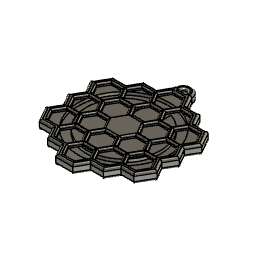
Base-v02 v3 (Autodesk Fusion 360 design; units mm, degrees)
Autodesk Fusion 360 part; units mm, degrees
note: some values were not read from the file. Set by a fixed rule: which sketch regions a step uses.
(part 1 of 2)
sketch "Skizze1" plane through (0, 0, 0) normal (0, 0, 1) x (1, 0, 0)
  line L0 (2.1651, -11.25) -> (4.3301, -7.5) construction
  line L1 (4.3301, -7.5) -> (2.1651, -3.75) construction
  line L2 (2.1651, -3.75) -> (-2.1651, -3.75) construction
  line L3 (-2.1651, -3.75) -> (-4.3301, -7.5) construction
  line L4 (-4.3301, -7.5) -> (-2.1651, -11.25) construction
  line L5 (-2.1651, -11.25) -> (2.1651, -11.25) construction
  line L6 (-2.1651, -3.75) -> (-4.3301, 0) construction
  line L7 (-4.3301, 0) -> (-8.6603, 0) construction
  line L8 (-8.6603, 0) -> (-10.8253, -3.75) construction
  line L9 (-10.8253, -3.75) -> (-8.6603, -7.5) construction
  line L10 (-8.6603, -7.5) -> (-4.3301, -7.5) construction
  line L11 (-4.3301, -7.5) -> (-2.1651, -3.75) construction
  line L12 (-4.3301, -7.5) -> (-8.6603, -7.5) construction
  line L13 (-8.6603, -7.5) -> (-10.8253, -11.25) construction
  line L14 (-10.8253, -11.25) -> (-8.6603, -15) construction
  line L15 (-8.6603, -15) -> (-4.3301, -15) construction
  line L16 (-4.3301, -15) -> (-2.1651, -11.25) construction
  line L17 (-2.1651, -11.25) -> (-4.3301, -7.5) construction
  line L18 (10.8253, -11.25) -> (8.6603, -7.5) construction
  line L19 (8.6603, -7.5) -> (4.3301, -7.5) construction
  line L20 (4.3301, -7.5) -> (2.1651, -11.25) construction
  line L21 (2.1651, -11.25) -> (4.3301, -15) construction
  line L22 (4.3301, -15) -> (8.6603, -15) construction
  line L23 (8.6603, -15) -> (10.8253, -11.25) construction
  line L24 (10.8253, -3.75) -> (8.6603, 0) construction
  line L25 (8.6603, 0) -> (4.3301, 0) construction
  line L26 (4.3301, 0) -> (2.1651, -3.75) construction
  line L27 (2.1651, -3.75) -> (4.3301, -7.5) construction
  line L28 (4.3301, -7.5) -> (8.6603, -7.5) construction
  line L29 (8.6603, -7.5) -> (10.8253, -3.75) construction
  line L30 (17.3205, 0) -> (15.1554, 3.75) construction
  line L31 (15.1554, 3.75) -> (10.8253, 3.75) construction
  line L32 (10.8253, 3.75) -> (8.6603, 0) construction
  line L33 (8.6603, 0) -> (10.8253, -3.75) construction
  line L34 (10.8253, -3.75) -> (15.1554, -3.75) construction
  line L35 (15.1554, -3.75) -> (17.3205, 0) construction
  line L36 (8.6603, -7.5) -> (10.8253, -11.25) construction
  line L37 (10.8253, -11.25) -> (15.1554, -11.25) construction
  line L38 (15.1554, -11.25) -> (17.3205, -7.5) construction
  line L39 (17.3205, -7.5) -> (15.1554, -3.75) construction
  line L40 (15.1554, -3.75) -> (10.8253, -3.75) construction
  line L41 (10.8253, -3.75) -> (8.6603, -7.5) construction
  line L42 (-4.3301, 0) -> (-2.1651, -3.75) construction
  line L43 (-2.1651, -3.75) -> (2.1651, -3.75) construction
  line L44 (2.1651, -3.75) -> (4.3301, 0) construction
  line L45 (4.3301, 0) -> (2.1651, 3.75) construction
  line L46 (2.1651, 3.75) -> (-2.1651, 3.75) construction
  line L47 (-2.1651, 3.75) -> (-4.3301, 0) construction
  line L48 (-8.6603, -22.5) -> (-4.3301, -22.5) construction
  line L49 (-4.3301, -22.5) -> (-2.1651, -18.75) construction
  line L50 (-2.1651, -18.75) -> (-4.3301, -15) construction
  line L51 (-4.3301, -15) -> (-8.6603, -15) construction
  line L52 (-8.6603, -15) -> (-10.8253, -18.75) construction
  line L53 (-10.8253, -18.75) -> (-8.6603, -22.5) construction
  line L54 (8.6603, -30) -> (10.8253, -26.25) construction
  line L55 (10.8253, -26.25) -> (8.6603, -22.5) construction
  line L56 (8.6603, -22.5) -> (4.3301, -22.5) construction
  line L57 (4.3301, -22.5) -> (2.1651, -26.25) construction
  line L58 (2.1651, -26.25) -> (4.3301, -30) construction
  line L59 (4.3301, -30) -> (8.6603, -30) construction
  line L60 (2.1651, -26.25) -> (4.3301, -22.5) construction
  line L61 (4.3301, -22.5) -> (2.1651, -18.75) construction
  line L62 (2.1651, -18.75) -> (-2.1651, -18.75) construction
  line L63 (-2.1651, -18.75) -> (-4.3301, -22.5) construction
  line L64 (-4.3301, -22.5) -> (-2.1651, -26.25) construction
  line L65 (-2.1651, -26.25) -> (2.1651, -26.25) construction
  line L66 (23.8157, -11.25) -> (21.6506, -7.5) construction
  line L67 (21.6506, -7.5) -> (17.3205, -7.5) construction
  line L68 (17.3205, -7.5) -> (15.1554, -11.25) construction
  line L69 (15.1554, -11.25) -> (17.3205, -15) construction
  line L70 (17.3205, -15) -> (21.6506, -15) construction
  line L71 (21.6506, -15) -> (23.8157, -11.25) construction
  line L72 (10.8253, -18.75) -> (8.6603, -15) construction
  line L73 (8.6603, -15) -> (4.3301, -15) construction
  line L74 (4.3301, -15) -> (2.1651, -18.75) construction
  line L75 (2.1651, -18.75) -> (4.3301, -22.5) construction
  line L76 (4.3301, -22.5) -> (8.6603, -22.5) construction
  line L77 (8.6603, -22.5) -> (10.8253, -18.75) construction
  line L78 (15.1554, -18.75) -> (10.8253, -18.75) construction
  line L79 (10.8253, -18.75) -> (8.6603, -22.5) construction
  line L80 (8.6603, -22.5) -> (10.8253, -26.25) construction
  line L81 (10.8253, -26.25) -> (15.1554, -26.25) construction
  line L82 (15.1554, -26.25) -> (17.3205, -22.5) construction
  line L83 (17.3205, -22.5) -> (15.1554, -18.75) construction
  line L84 (8.6603, 7.5) -> (4.3301, 7.5) construction
  line L85 (4.3301, 7.5) -> (2.1651, 3.75) construction
  line L86 (2.1651, 3.75) -> (4.3301, 0) construction
  line L87 (4.3301, 0) -> (8.6603, 0) construction
  line L88 (8.6603, 0) -> (10.8253, 3.75) construction
  line L89 (10.8253, 3.75) -> (8.6603, 7.5) construction
  line L90 (15.1554, -11.25) -> (10.8253, -11.25) construction
  line L91 (10.8253, -11.25) -> (8.6603, -15) construction
  line L92 (8.6603, -15) -> (10.8253, -18.75) construction
  line L93 (10.8253, -18.75) -> (15.1554, -18.75) construction
  line L94 (15.1554, -18.75) -> (17.3205, -15) construction
  line L95 (17.3205, -15) -> (15.1554, -11.25) construction
  line L96 (21.6506, 0) -> (17.3205, 0) construction
  line L97 (17.3205, 0) -> (15.1554, -3.75) construction
  line L98 (15.1554, -3.75) -> (17.3205, -7.5) construction
  line L99 (17.3205, -7.5) -> (21.6506, -7.5) construction
  line L100 (21.6506, -7.5) -> (23.8157, -3.75) construction
  line L101 (23.8157, -3.75) -> (21.6506, 0) construction
  line L102 (2.1651, -18.75) -> (4.3301, -15) construction
  line L103 (4.3301, -15) -> (2.1651, -11.25) construction
  line L104 (2.1651, -11.25) -> (-2.1651, -11.25) construction
  line L105 (-2.1651, -11.25) -> (-4.3301, -15) construction
  line L106 (-4.3301, -15) -> (-2.1651, -18.75) construction
  line L107 (-2.1651, -18.75) -> (2.1651, -18.75) construction
  line L108 (23.8157, -18.75) -> (21.6506, -15) construction
  line L109 (21.6506, -15) -> (17.3205, -15) construction
  line L110 (17.3205, -15) -> (15.1554, -18.75) construction
  line L111 (15.1554, -18.75) -> (17.3205, -22.5) construction
  line L112 (17.3205, -22.5) -> (21.6506, -22.5) construction
  line L113 (21.6506, -22.5) -> (23.8157, -18.75) construction
  line L114 (4.6765, 0.6) -> (8.3138, 0.6)
  line L115 (8.3138, 0.6) -> (10.1325, 3.75)
  line L116 (10.1325, 3.75) -> (8.3138, 6.9)
  line L117 (8.3138, 6.9) -> (4.6765, 6.9)
  line L118 (4.6765, 6.9) -> (2.8579, 3.75)
  line L119 (2.8579, 3.75) -> (4.6765, 0.6)
  line L120 (14.809, -3.15) -> (16.6277, 0)
  line L121 (16.6277, 0) -> (14.809, 3.15)
  line L122 (14.809, 3.15) -> (11.1717, 3.15)
  line L123 (11.1717, 3.15) -> (9.3531, 0)
  line L124 (9.3531, 0) -> (11.1717, -3.15)
  line L125 (11.1717, -3.15) -> (14.809, -3.15)
  line L126 (21.3042, -6.9) -> (23.1229, -3.75)
  line L127 (23.1229, -3.75) -> (21.3042, -0.6)
  line L128 (21.3042, -0.6) -> (17.6669, -0.6)
  line L129 (17.6669, -0.6) -> (15.8483, -3.75)
  line L130 (15.8483, -3.75) -> (17.6669, -6.9)
  line L131 (17.6669, -6.9) -> (21.3042, -6.9)
  line L132 (14.809, -10.65) -> (16.6277, -7.5)
  line L133 (16.6277, -7.5) -> (14.809, -4.35)
  line L134 (14.809, -4.35) -> (11.1717, -4.35)
  line L135 (11.1717, -4.35) -> (9.3531, -7.5)
  line L136 (9.3531, -7.5) -> (11.1717, -10.65)
  line L137 (11.1717, -10.65) -> (14.809, -10.65)
  line L138 (15.8483, -11.25) -> (17.6669, -14.4)
  line L139 (17.6669, -14.4) -> (21.3042, -14.4)
  line L140 (21.3042, -14.4) -> (23.1229, -11.25)
  line L141 (23.1229, -11.25) -> (21.3042, -8.1)
  line L142 (21.3042, -8.1) -> (17.6669, -8.1)
  line L143 (17.6669, -8.1) -> (15.8483, -11.25)
  line L144 (11.1717, -18.15) -> (14.809, -18.15)
  line L145 (14.809, -18.15) -> (16.6277, -15)
  line L146 (16.6277, -15) -> (14.809, -11.85)
  line L147 (14.809, -11.85) -> (11.1717, -11.85)
  line L148 (11.1717, -11.85) -> (9.3531, -15)
  line L149 (9.3531, -15) -> (11.1717, -18.15)
  line L150 (-1.8187, -10.65) -> (1.8187, -10.65)
  line L151 (1.8187, -10.65) -> (3.6373, -7.5)
  line L152 (3.6373, -7.5) -> (1.8187, -4.35)
  line L153 (1.8187, -4.35) -> (-1.8187, -4.35)
  line L154 (-1.8187, -4.35) -> (-3.6373, -7.5)
  line L155 (-3.6373, -7.5) -> (-1.8187, -10.65)
  line L156 (-1.8187, -3.15) -> (1.8187, -3.15)
  line L157 (1.8187, -3.15) -> (3.6373, 0)
  line L158 (3.6373, 0) -> (1.8187, 3.15)
  line L159 (1.8187, 3.15) -> (-1.8187, 3.15)
  line L160 (-1.8187, 3.15) -> (-3.6373, 0)
  line L161 (-3.6373, 0) -> (-1.8187, -3.15)
  line L162 (-8.3138, -6.9) -> (-4.6765, -6.9)
  line L163 (-4.6765, -6.9) -> (-2.8579, -3.75)
  line L164 (-2.8579, -3.75) -> (-4.6765, -0.6)
  line L165 (-4.6765, -0.6) -> (-8.3138, -0.6)
  line L166 (-8.3138, -0.6) -> (-10.1325, -3.75)
  line L167 (-10.1325, -3.75) -> (-8.3138, -6.9)
  line L168 (-0.0476, -15) -> (-0.0238, -15.0412)
  line L169 (-0.0238, -15.0412) -> (0.0238, -15.0412)
  line L170 (0.0238, -15.0412) -> (0.0476, -15)
  line L171 (0.0476, -15) -> (0.0238, -14.9588)
  line L172 (0.0238, -14.9588) -> (-0.0238, -14.9588)
  line L173 (-0.0238, -14.9588) -> (-0.0476, -15)
  line L174 (10.1325, -18.75) -> (8.3138, -15.6)
  line L175 (8.3138, -15.6) -> (4.6765, -15.6)
  line L176 (4.6765, -15.6) -> (2.8579, -18.75)
  line L177 (2.8579, -18.75) -> (4.6765, -21.9)
  line L178 (4.6765, -21.9) -> (8.3138, -21.9)
  line L179 (8.3138, -21.9) -> (10.1325, -18.75)
  line L180 (23.1229, -18.75) -> (21.3042, -15.6)
  line L181 (21.3042, -15.6) -> (17.6669, -15.6)
  line L182 (17.6669, -15.6) -> (15.8483, -18.75)
  line L183 (15.8483, -18.75) -> (17.6669, -21.9)
  line L184 (17.6669, -21.9) -> (21.3042, -21.9)
  line L185 (21.3042, -21.9) -> (23.1229, -18.75)
  line L186 (8.3138, -6.9) -> (10.1325, -3.75)
  line L187 (10.1325, -3.75) -> (8.3138, -0.6)
  line L188 (8.3138, -0.6) -> (4.6765, -0.6)
  line L189 (4.6765, -0.6) -> (2.8579, -3.75)
  line L190 (2.8579, -3.75) -> (4.6765, -6.9)
  line L191 (4.6765, -6.9) -> (8.3138, -6.9)
  line L192 (-4.6765, -21.9) -> (-2.8579, -18.75)
  line L193 (-2.8579, -18.75) -> (-4.6765, -15.6)
  line L194 (-4.6765, -15.6) -> (-8.3138, -15.6)
  line L195 (-8.3138, -15.6) -> (-10.1325, -18.75)
  line L196 (-10.1325, -18.75) -> (-8.3138, -21.9)
  line L197 (-8.3138, -21.9) -> (-4.6765, -21.9)
  line L198 (1.8187, -25.65) -> (3.6373, -22.5)
  line L199 (3.6373, -22.5) -> (1.8187, -19.35)
  line L200 (1.8187, -19.35) -> (-1.8187, -19.35)
  line L201 (-1.8187, -19.35) -> (-3.6373, -22.5)
  line L202 (-3.6373, -22.5) -> (-1.8187, -25.65)
  line L203 (-1.8187, -25.65) -> (1.8187, -25.65)
  line L204 (10.1325, -26.25) -> (8.3138, -23.1)
  line L205 (8.3138, -23.1) -> (4.6765, -23.1)
  line L206 (4.6765, -23.1) -> (2.8579, -26.25)
  line L207 (2.8579, -26.25) -> (4.6765, -29.4)
  line L208 (4.6765, -29.4) -> (8.3138, -29.4)
  line L209 (8.3138, -29.4) -> (10.1325, -26.25)
  line L210 (16.6277, -22.5) -> (14.809, -19.35)
  line L211 (14.809, -19.35) -> (11.1717, -19.35)
  line L212 (11.1717, -19.35) -> (9.3531, -22.5)
  line L213 (9.3531, -22.5) -> (11.1717, -25.65)
  line L214 (11.1717, -25.65) -> (14.809, -25.65)
  line L215 (14.809, -25.65) -> (16.6277, -22.5)
  line L216 (-1.8187, -18.15) -> (1.8187, -18.15)
  line L217 (1.8187, -18.15) -> (3.6373, -15)
  line L218 (3.6373, -15) -> (1.8187, -11.85)
  line L219 (1.8187, -11.85) -> (-1.8187, -11.85)
  line L220 (-1.8187, -11.85) -> (-3.6373, -15)
  line L221 (-3.6373, -15) -> (-1.8187, -18.15)
  line L222 (-8.3138, -14.4) -> (-4.6765, -14.4)
  line L223 (-4.6765, -14.4) -> (-2.8579, -11.25)
  line L224 (-2.8579, -11.25) -> (-4.6765, -8.1)
  line L225 (-4.6765, -8.1) -> (-8.3138, -8.1)
  line L226 (-8.3138, -8.1) -> (-10.1325, -11.25)
  line L227 (-10.1325, -11.25) -> (-8.3138, -14.4)
  line L228 (11.5181, 4.95) -> (9.3531, 8.7)
  line L229 (9.3531, 8.7) -> (3.6373, 8.7)
  line L230 (3.6373, 8.7) -> (1.4722, 4.95)
  line L231 (1.4722, 4.95) -> (-2.8579, 4.95)
  line L232 (-2.8579, 4.95) -> (-5.0229, 1.2)
  line L233 (-5.0229, 1.2) -> (-9.3531, 1.2)
  line L234 (-9.3531, 1.2) -> (-12.211, -3.75)
  line L235 (-12.211, -3.75) -> (-10.0459, -7.5)
  line L236 (-10.0459, -7.5) -> (-12.211, -11.25)
  line L237 (-12.211, -11.25) -> (-10.0459, -15)
  line L238 (-10.0459, -15) -> (-12.211, -18.75)
  line L239 (-12.211, -18.75) -> (-9.3531, -23.7)
  line L240 (-9.3531, -23.7) -> (-5.0229, -23.7)
  line L241 (-5.0229, -23.7) -> (-2.8579, -27.45)
  line L242 (-2.8579, -27.45) -> (1.4722, -27.45)
  line L243 (1.4722, -27.45) -> (3.6373, -31.2)
  line L244 (3.6373, -31.2) -> (9.3531, -31.2)
  line L245 (9.3531, -31.2) -> (11.5181, -27.45)
  line L246 (11.5181, -27.45) -> (15.8483, -27.45)
  line L247 (15.8483, -27.45) -> (18.0133, -23.7)
  line L248 (18.0133, -23.7) -> (22.3435, -23.7)
  line L249 (22.3435, -23.7) -> (25.2013, -18.75)
  line L250 (25.2013, -18.75) -> (23.0363, -15)
  line L251 (23.0363, -15) -> (25.2013, -11.25)
  line L252 (25.2013, -11.25) -> (23.0363, -7.5)
  line L253 (23.0363, -7.5) -> (25.2013, -3.75)
  line L254 (25.2013, -3.75) -> (22.3435, 1.2)
  line L255 (22.3435, 1.2) -> (18.0133, 1.2)
  line L256 (18.0133, 1.2) -> (15.8483, 4.95)
  line L257 (15.8483, 4.95) -> (11.5181, 4.95)
  arc A0 (9.3531, 8.7) -> (3.6373, 8.7) centre (6.4952, 8.7) ccw
  arc A1 (7.5531, 8.7) -> (5.4373, 8.7) centre (6.4952, 8.7) ccw
  point P0 (0, -7.5)
  point P1 (-6.4952, -3.75)
  point P2 (-6.4952, -11.25)
  point P3 (6.4952, -11.25)
  point P4 (6.4952, -3.75)
  point P5 (12.9904, 0)
  point P6 (12.9904, -7.5)
  point P7 (-6.4952, -18.75)
  point P8 (6.4952, -26.25)
  point P9 (0, -22.5)
  point P10 (19.4856, -11.25)
  point P11 (6.4952, -18.75)
  point P12 (12.9904, -22.5)
  point P13 (6.4952, 3.75)
  point P14 (12.9904, -15)
  point P15 (19.4856, -3.75)
  point P16 (0, -15)
  point P17 (19.4856, -18.75)
  point P18 (6.4952, 3.75)
  point P19 (12.9904, 0)
  point P20 (19.4856, -3.75)
  point P21 (12.9904, -7.5)
  point P22 (19.4856, -11.25)
  point P23 (12.9904, -15)
  point P24 (6.4952, -11.25)
  point P25 (0, -7.5)
  point P26 (-6.4952, -3.75)
  point P27 (-6.4952, -11.25)
  point P28 (0, -15)
  point P29 (6.4952, -18.75)
  point P30 (19.4856, -18.75)
  point P31 (6.4952, -3.75)
  point P32 (-6.4952, -18.75)
  point P33 (0, -22.5)
  point P34 (6.4952, -26.25)
  point P35 (12.9904, -22.5)
  point P36 (0, -15)
  point P37 (-6.4952, -11.25)
  point P38 (6.4952, 8.7)
  point P39 (6.4952, 6.9)
  dimension "d1" = 7.5
  dimension "d2" = 6.3
  dimension "d3" = 1.2
  dimension "d8" = 39.9
  dimension "d9" = -1.8
  constraint horizontal L2
  constraint equal L40 L45
  constraint equal L32 L45
  constraint equal L26 L40
  constraint equal L2 L40
  constraint equal L19 L40
  constraint equal L13 L46
  constraint equal L7 L46
  constraint equal L46 L103
  constraint equal L46 L55
  constraint equal L46 L50
  constraint equal L45 L61
  constraint equal L44 L67
  constraint equal L44 L73
  constraint equal L44 L79
  constraint equal L44 L85
  constraint equal L44 L91
  constraint equal L44 L97
  constraint horizontal L51
  constraint horizontal L46
  constraint horizontal L40
  constraint horizontal L31
  constraint horizontal L25
  constraint horizontal L7
  constraint horizontal L56
  constraint horizontal L104
  constraint horizontal L19
  constraint horizontal L96
  constraint horizontal L90
  constraint horizontal L84
  constraint horizontal L78
  constraint horizontal L73
  constraint horizontal L67
  constraint horizontal L62
  constraint midpoint L6 L42
  constraint midpoint L2 L43
  constraint midpoint L26 L44
  constraint midpoint L29 L41
  constraint midpoint L19 L28
  constraint midpoint L34 L40
  constraint midpoint L35 L97
  constraint midpoint L37 L90
  constraint midpoint L5 L104
  constraint midpoint L22 L73
  constraint horizontal L12
  constraint midpoint L10 L12
  constraint midpoint L25 L87
  constraint midpoint L15 L51
  constraint midpoint L62 L107
  constraint midpoint L56 L76
  constraint midpoint L78 L93
  constraint midpoint L67 L99
  constraint equal L46 L109
  constraint horizontal L109
  constraint midpoint L70 L109
  constraint coincident P18 P13
  constraint coincident P19 P5
  constraint coincident P20 P15
  constraint coincident P21 P6
  constraint coincident P22 P10
  constraint coincident P23 P14
  constraint coincident P24 P3
  constraint coincident P25 P0
  constraint coincident P26 P1
  constraint coincident P37 P27
  constraint coincident P36 P28
  constraint coincident P29 P11
  constraint coincident P30 P17
  constraint coincident P31 P4
  constraint coincident P32 P7
  constraint coincident P33 P9
  constraint coincident P34 P8
  constraint coincident P35 P12
  constraint horizontal L117
  constraint horizontal L122
  constraint horizontal L128
  constraint horizontal L134
  constraint horizontal L142
  constraint horizontal L181
  constraint horizontal L147
  constraint horizontal L211
  constraint horizontal L205
  constraint horizontal L175
  constraint horizontal L188
  constraint horizontal L153
  constraint horizontal L169
  constraint horizontal L200
  constraint horizontal L194
  constraint horizontal L165
  constraint horizontal L219
  constraint horizontal L225
  constraint horizontal L159
  constraint equal L117 L122
  constraint equal L122 L159
  constraint equal L114 L188
  constraint equal L120 L128
  constraint equal L125 L134
  constraint equal L131 L142
  constraint equal L137 L147
  constraint equal L152 L190
  constraint equal L161 L164
  constraint equal L162 L225
  constraint equal L150 L219
  constraint equal L194 L222
  constraint equal L200 L216
  constraint equal L178 L205
  constraint equal L144 L211
  constraint equal L139 L181
  constraint equal L175 L188
  constraint midpoint L117 P39
  constraint midpoint L229 P38
  constraint coincident P38 A0.centre
  measures "d1" distance of L42 L45
  measures "d2" distance of L116 L119
  measures "d8" distance of L229 L244
extrude "Extrusion1" add sketch "Skizze1" along normal blind 1 contours L228 L229 L230 L231 L232 L233 L234 L235 L236 L237 L238 L239 L240 L241 L242 L243 L244 L245 L246 L247 L248 L249 L250 L251 L252 L253 L254 L255 L256 L257 | L229 A0 A1
sketch "Skizze2" plane through (0, 0, 0) normal (0, 0, -1) x (1, 0, 0)
  line L0 (-8.6603, 7.5) -> (-10.8253, 3.75) construction
  line L1 (-10.0459, 7.5) -> (-12.211, 3.75)
  line L2 (-8.3138, 8.1) -> (-4.6765, 8.1) construction
  line L3 (-12.211, 11.25) -> (-10.0459, 7.5)
  line L4 (21.3042, 8.1) -> (23.1229, 11.25) construction
  line L5 (10.8253, 11.25) -> (15.1554, 11.25) construction
  line L6 (15.1554, 3.75) -> (17.3205, 7.5) construction
  line L7 (23.8157, 3.75) -> (21.6506, 7.5) construction
  line L8 (9.3531, 7.5) -> (11.1717, 4.35) construction
  line L9 (15.1554, 3.75) -> (10.8253, 3.75) construction
  line L10 (15.1554, 11.25) -> (17.3205, 7.5) construction
  line L11 (21.6506, 7.5) -> (17.3205, 7.5) construction
  line L12 (17.6669, 6.9) -> (15.8483, 3.75) construction
  line L13 (-8.6603, 7.5) -> (-4.3301, 7.5) construction
  line L14 (1.4722, -4.95) -> (3.6373, -8.7)
  line L15 (1.8187, 19.35) -> (3.6373, 22.5) construction
  line L16 (-8.6603, 0) -> (-4.3301, 0) construction
  line L17 (1.8187, 3.15) -> (-1.8187, 3.15) construction
  line L18 (4.3301, 7.5) -> (2.1651, 11.25) construction
  line L19 (2.8579, 18.75) -> (4.6765, 15.6) construction
  line L20 (-1.8187, 11.85) -> (1.8187, 11.85) construction
  line L21 (-10.1325, 11.25) -> (-8.3138, 8.1) construction
  line L22 (21.3042, 14.4) -> (17.6669, 14.4) construction
  line L23 (2.1651, -3.75) -> (4.3301, -7.5) construction
  line L24 (17.3205, 15) -> (21.6506, 15) construction
  line L25 (-1.8187, 18.15) -> (-3.6373, 15) construction
  line L26 (8.3138, 15.6) -> (10.1325, 18.75) construction
  line L27 (11.1717, 11.85) -> (14.809, 11.85) construction
  line L28 (-2.8579, -4.95) -> (1.4722, -4.95)
  line L29 (21.6506, 22.5) -> (17.3205, 22.5) construction
  line L30 (22.3435, 23.7) -> (18.0133, 23.7)
  line L31 (23.8157, 18.75) -> (21.6506, 22.5) construction
  line L32 (2.1651, 3.75) -> (-2.1651, 3.75) construction
  line L33 (1.8187, 11.85) -> (3.6373, 15) construction
  line L34 (-2.1651, 18.75) -> (-4.3301, 15) construction
  line L35 (-8.3138, 6.9) -> (-10.1325, 3.75) construction
  line L36 (-10.8253, 11.25) -> (-8.6603, 7.5) construction
  line L37 (2.1651, 18.75) -> (-2.1651, 18.75) construction
  line L38 (4.6765, -0.6) -> (2.8579, -3.75) construction
  line L39 (2.1651, 26.25) -> (4.3301, 22.5) construction
  line L40 (-4.3301, 15) -> (-2.1651, 18.75) construction
  line L41 (3.6373, 15) -> (1.8187, 18.15) construction
  line L42 (-5.0229, -1.2) -> (-2.8579, -4.95)
  line L43 (-1.8187, -3.15) -> (1.8187, -3.15) construction
  line L44 (-3.6373, 22.5) -> (-1.8187, 19.35) construction
  line L45 (-2.8579, 3.75) -> (-4.6765, 6.9) construction
  line L46 (21.3042, 21.9) -> (17.6669, 21.9) construction
  line L47 (1.8187, 10.65) -> (-1.8187, 10.65) construction
  line L48 (-4.3301, 7.5) -> (-2.1651, 3.75) construction
  line L49 (-4.3301, 7.5) -> (-2.1651, 11.25) construction
  line L50 (-2.1651, 11.25) -> (2.1651, 11.25) construction
  line L51 (25.2013, 18.75) -> (22.3435, 23.7)
  line L52 (1.8187, 25.65) -> (-1.8187, 25.65) construction
  line L53 (2.1651, 11.25) -> (-2.1651, 11.25) construction
  line L54 (-4.3301, 7.5) -> (-8.6603, 7.5) construction
  line L55 (-4.6765, 6.9) -> (-8.3138, 6.9) construction
  line L56 (-8.3138, 0.6) -> (-4.6765, 0.6) construction
  line L57 (23.1229, 18.75) -> (21.3042, 21.9) construction
  line L58 (4.3301, 22.5) -> (2.1651, 18.75) construction
  line L59 (1.8187, 18.15) -> (-1.8187, 18.15) construction
  line L60 (-9.3531, -1.2) -> (-5.0229, -1.2)
  line L61 (-2.1651, 3.75) -> (2.1651, 3.75) construction
  line L62 (21.3042, 15.6) -> (23.1229, 18.75) construction
  line L63 (10.8253, 18.75) -> (8.6603, 22.5) construction
  line L64 (21.6506, 15) -> (23.8157, 18.75) construction
  line L65 (-1.8187, 4.35) -> (1.8187, 4.35) construction
  line L66 (9.3531, 22.5) -> (11.1717, 19.35) construction
  line L67 (3.6373, 22.5) -> (1.8187, 25.65) construction
  line L68 (4.3301, 0) -> (2.1651, -3.75) construction
  line L69 (-2.1651, 26.25) -> (-4.3301, 22.5) construction
  line L70 (1.8187, 4.35) -> (3.6373, 7.5) construction
  line L71 (12.9666, 14.9588) -> (13.0142, 14.9588) construction
  line L72 (14.809, 11.85) -> (16.6277, 15) construction
  line L73 (-2.1651, 18.75) -> (2.1651, 18.75) construction
  line L74 (2.1651, -3.75) -> (4.3301, 0) construction
  line L75 (13.0142, 15.0412) -> (12.9666, 15.0412) construction
  line L76 (-4.3301, 22.5) -> (-2.1651, 18.75) construction
  line L77 (-2.1651, -3.75) -> (2.1651, -3.75) construction
  line L78 (4.3301, 15) -> (2.1651, 18.75) construction
  line L79 (14.809, 18.15) -> (11.1717, 18.15) construction
  line L80 (3.6373, 31.2) -> (1.4722, 27.45)
  line L81 (-1.8187, 10.65) -> (-3.6373, 7.5) construction
  line L82 (17.6669, 15.6) -> (21.3042, 15.6) construction
  line L83 (10.1325, 18.75) -> (8.3138, 21.9) construction
  line L84 (13.0142, 14.9588) -> (13.038, 15) construction
  line L85 (-4.3301, 0) -> (-2.1651, -3.75) construction
  line L86 (23.0363, 15) -> (25.2013, 18.75)
  line L87 (-2.1651, 18.75) -> (-4.3301, 22.5) construction
  line L88 (4.3301, 7.5) -> (2.1651, 3.75) construction
  line L89 (21.6506, 15) -> (17.3205, 15) construction
  line L90 (-4.6765, 8.1) -> (-2.8579, 11.25) construction
  line L91 (2.1651, 18.75) -> (4.3301, 22.5) construction
  line L92 (-2.1651, 3.75) -> (-4.3301, 7.5) construction
  line L93 (2.1651, 3.75) -> (4.3301, 7.5) construction
  line L94 (-3.6373, 0) -> (-1.8187, -3.15) construction
  line L95 (2.8579, -3.75) -> (4.6765, -6.9) construction
  line L96 (12.9666, 15.0412) -> (12.9428, 15) construction
  line L97 (15.1554, 18.75) -> (10.8253, 18.75) construction
  line L98 (3.6373, 7.5) -> (1.8187, 10.65) construction
  line L99 (10.8253, 18.75) -> (15.1554, 18.75) construction
  line L100 (10.8253, 18.75) -> (8.6603, 15) construction
  line L101 (1.8187, -3.15) -> (3.6373, 0) construction
  line L102 (4.3301, 22.5) -> (2.1651, 26.25) construction
  line L103 (2.1651, 11.25) -> (4.3301, 7.5) construction
  line L104 (-3.6373, 15) -> (-1.8187, 11.85) construction
  line L105 (25.2013, 11.25) -> (23.0363, 15)
  line L106 (16.6277, 7.5) -> (14.809, 10.65) construction
  line L107 (17.6669, 8.1) -> (21.3042, 8.1) construction
  line L108 (10.8253, 11.25) -> (8.6603, 7.5) construction
  line L109 (21.3042, 6.9) -> (17.6669, 6.9) construction
  line L110 (10.1325, 3.75) -> (8.3138, 6.9) construction
  line L111 (21.6506, 7.5) -> (23.8157, 11.25) construction
  line L112 (11.1717, 10.65) -> (9.3531, 7.5) construction
  line L113 (15.8483, 11.25) -> (17.6669, 8.1) construction
  line L114 (17.3205, 7.5) -> (21.6506, 7.5) construction
  line L115 (17.3205, 7.5) -> (15.1554, 11.25) construction
  line L116 (-10.0459, 15) -> (-12.211, 11.25)
  line L117 (15.1554, 11.25) -> (10.8253, 11.25) construction
  line L118 (10.8253, 3.75) -> (15.1554, 3.75) construction
  line L119 (-2.1651, 11.25) -> (-4.3301, 15) construction
  line L120 (10.8253, 3.75) -> (8.6603, 7.5) construction
  line L121 (8.6603, 7.5) -> (10.8253, 3.75) construction
  line L122 (14.809, 4.35) -> (16.6277, 7.5) construction
  line L123 (17.3205, 7.5) -> (15.1554, 3.75) construction
  line L124 (23.0363, 7.5) -> (25.2013, 11.25)
  line L125 (23.1229, 3.75) -> (21.3042, 6.9) construction
  line L126 (11.1717, 4.35) -> (14.809, 4.35) construction
  line L127 (8.6603, 7.5) -> (10.8253, 11.25) construction
  line L128 (14.809, 10.65) -> (11.1717, 10.65) construction
  line L129 (25.2013, 3.75) -> (23.0363, 7.5)
  line L130 (8.6603, 7.5) -> (4.3301, 7.5) construction
  arc A0 (3.6373, -8.7) -> (9.3531, -8.7) centre (6.4952, -8.7) ccw
  line L131 (-2.8579, 18.75) -> (-4.6765, 21.9) construction
  line L132 (-4.3301, 15) -> (-8.6603, 15) construction
  line L133 (4.3301, -7.5) -> (8.6603, -7.5) construction
  line L134 (8.3138, 21.9) -> (4.6765, 21.9) construction
  line L135 (11.1717, 25.65) -> (9.3531, 22.5) construction
  line L136 (17.3205, 22.5) -> (15.1554, 26.25) construction
  line L137 (8.6603, 15) -> (4.3301, 15) construction
  line L138 (10.8253, -3.75) -> (15.1554, -3.75) construction
  line L139 (8.6603, 30) -> (4.3301, 30) construction
  line L140 (8.3138, 29.4) -> (4.6765, 29.4) construction
  line L141 (18.0133, 23.7) -> (15.8483, 27.45)
  line L142 (21.3042, 0.6) -> (23.1229, 3.75) construction
  line L143 (-10.8253, 3.75) -> (-8.6603, 0) construction
  line L144 (-4.6765, 0.6) -> (-2.8579, 3.75) construction
  line L145 (15.1554, 3.75) -> (17.3205, 0) construction
  line L146 (9.3531, 31.2) -> (3.6373, 31.2)
  line L147 (15.8483, 3.75) -> (17.6669, 0.6) construction
  line L148 (2.8579, 3.75) -> (4.6765, 0.6) construction
  line L149 (4.6765, 23.1) -> (8.3138, 23.1) construction
  line L150 (4.6765, 15.6) -> (8.3138, 15.6) construction
  line L151 (8.6603, 0) -> (4.3301, 0) construction
  line L152 (8.6603, 22.5) -> (10.8253, 26.25) construction
  line L153 (-4.3301, 22.5) -> (-8.6603, 22.5) construction
  line L154 (8.3138, 6.9) -> (4.6765, 6.9) construction
  line L155 (21.6506, 0) -> (23.8157, 3.75) construction
  line L156 (17.3205, 0) -> (15.1554, 3.75) construction
  line L157 (15.8483, 27.45) -> (11.5181, 27.45)
  line L158 (10.1325, 26.25) -> (8.3138, 29.4) construction
  line L159 (15.1554, 18.75) -> (17.3205, 15) construction
  arc A1 (5.4373, -8.7) -> (7.5531, -8.7) centre (6.4952, -8.7) ccw
  line L160 (-8.6603, 15) -> (-4.3301, 15) construction
  line L161 (22.3435, -1.2) -> (25.2013, 3.75)
  line L162 (11.1717, -3.15) -> (14.809, -3.15) construction
  line L163 (4.3301, 22.5) -> (8.6603, 22.5) construction
  line L164 (4.6765, -6.9) -> (8.3138, -6.9) construction
  line L165 (4.3301, 7.5) -> (8.6603, 7.5) construction
  line L166 (4.3301, 15) -> (8.6603, 15) construction
  line L167 (3.6373, -8.7) -> (9.3531, -8.7)
  line L168 (8.6603, 22.5) -> (4.3301, 22.5) construction
  line L169 (4.6765, 0.6) -> (8.3138, 0.6) construction
  line L170 (4.3301, 0) -> (8.6603, 0) construction
  line L171 (8.3138, 0.6) -> (10.1325, 3.75) construction
  line L172 (16.6277, 22.5) -> (14.809, 25.65) construction
  line L173 (10.8253, 26.25) -> (8.6603, 22.5) construction
  line L174 (-4.6765, 15.6) -> (-2.8579, 18.75) construction
  line L175 (8.3138, 23.1) -> (10.1325, 26.25) construction
  line L176 (8.3138, -0.6) -> (4.6765, -0.6) construction
  line L177 (8.6603, 0) -> (10.8253, 3.75) construction
  line L178 (10.8253, 3.75) -> (8.6603, 0) construction
  line L179 (-1.8187, 19.35) -> (1.8187, 19.35) construction
  line L180 (-5.0229, 23.7) -> (-9.3531, 23.7)
  line L181 (-10.1325, 18.75) -> (-8.3138, 15.6) construction
  line L182 (-12.211, 3.75) -> (-9.3531, -1.2)
  line L183 (-3.6373, 7.5) -> (-1.8187, 4.35) construction
  line L184 (2.1651, 26.25) -> (-2.1651, 26.25) construction
  line L185 (10.8253, 26.25) -> (8.6603, 30) construction
  line L186 (4.6765, 29.4) -> (2.8579, 26.25) construction
  line L187 (2.1651, 3.75) -> (4.3301, 0) construction
  line L188 (2.8579, 26.25) -> (4.6765, 23.1) construction
  line L189 (9.3531, 15) -> (11.1717, 11.85) construction
  line L190 (12.9428, 15) -> (12.9666, 14.9588) construction
  line L191 (2.1651, 18.75) -> (4.3301, 15) construction
  line L192 (8.6603, 15) -> (10.8253, 18.75) construction
  line L193 (-4.3301, 0) -> (-2.1651, 3.75) construction
  line L194 (15.1554, 18.75) -> (17.3205, 22.5) construction
  line L195 (-4.6765, 21.9) -> (-8.3138, 21.9) construction
  line L196 (-2.1651, 3.75) -> (-4.3301, 0) construction
  line L197 (4.3301, 30) -> (2.1651, 26.25) construction
  line L198 (16.6277, 15) -> (14.809, 18.15) construction
  line L199 (-2.1651, 11.25) -> (-4.3301, 7.5) construction
  line L200 (15.8483, 18.75) -> (17.6669, 15.6) construction
  line L201 (15.1554, 26.25) -> (10.8253, 26.25) construction
  line L202 (13.038, 15) -> (13.0142, 15.0412) construction
  line L203 (-8.6603, 22.5) -> (-10.8253, 18.75) construction
  line L204 (-4.6765, 14.4) -> (-8.3138, 14.4) construction
  line L205 (-1.8187, 3.15) -> (-3.6373, 0) construction
  line L206 (-10.8253, 18.75) -> (-8.6603, 15) construction
  line L207 (14.809, 19.35) -> (16.6277, 22.5) construction
  line L208 (4.3301, 0) -> (2.1651, 3.75) construction
  line L209 (-8.3138, 15.6) -> (-4.6765, 15.6) construction
  line L210 (-2.8579, 27.45) -> (-5.0229, 23.7)
  line L211 (17.6669, 21.9) -> (15.8483, 18.75) construction
  line L212 (-12.211, 18.75) -> (-10.0459, 15)
  line L213 (11.5181, 27.45) -> (9.3531, 31.2)
  line L214 (4.6765, 21.9) -> (2.8579, 18.75) construction
  line L215 (8.6603, 22.5) -> (10.8253, 18.75) construction
  line L216 (11.1717, 18.15) -> (9.3531, 15) construction
  line L217 (3.6373, 0) -> (1.8187, 3.15) construction
  line L218 (14.809, 25.65) -> (11.1717, 25.65) construction
  line L219 (17.3205, 22.5) -> (15.1554, 18.75) construction
  line L220 (-10.1325, 3.75) -> (-8.3138, 0.6) construction
  line L221 (11.1717, 19.35) -> (14.809, 19.35) construction
  line L222 (17.3205, 15) -> (15.1554, 18.75) construction
  line L223 (-1.8187, 25.65) -> (-3.6373, 22.5) construction
  line L224 (-9.3531, 23.7) -> (-12.211, 18.75)
  line L225 (-8.3138, 21.9) -> (-10.1325, 18.75) construction
  line L226 (4.6765, 6.9) -> (2.8579, 3.75) construction
  line L227 (1.4722, 27.45) -> (-2.8579, 27.45)
  line L228 (16.6277, 0) -> (14.809, 3.15) construction
  line L229 (-2.8579, 11.25) -> (-4.6765, 14.4) construction
  line L230 (8.6603, -7.5) -> (10.8253, -3.75) construction
  line L231 (17.3205, 0) -> (21.6506, 0) construction
  line L232 (23.8157, 11.25) -> (21.6506, 15) construction
  line L233 (14.809, -3.15) -> (16.6277, 0) construction
  line L234 (15.1554, 11.25) -> (17.3205, 15) construction
  line L235 (8.6603, 0) -> (10.8253, -3.75) construction
  line L236 (11.1717, 3.15) -> (9.3531, 0) construction
  line L237 (10.1325, -3.75) -> (8.3138, -0.6) construction
  line L238 (9.3531, -8.7) -> (11.5181, -4.95)
  line L239 (23.1229, 11.25) -> (21.3042, 14.4) construction
  line L240 (10.8253, 11.25) -> (8.6603, 15) construction
  line L241 (17.6669, 14.4) -> (15.8483, 11.25) construction
  line L242 (11.5181, -4.95) -> (15.8483, -4.95)
  line L243 (15.1554, -3.75) -> (17.3205, 0) construction
  line L244 (14.809, 3.15) -> (11.1717, 3.15) construction
  line L245 (2.1651, 11.25) -> (4.3301, 15) construction
  line L246 (4.3301, 15) -> (2.1651, 11.25) construction
  line L247 (-4.3301, 15) -> (-2.1651, 11.25) construction
  line L248 (9.3531, 0) -> (11.1717, -3.15) construction
  line L249 (17.3205, 15) -> (15.1554, 11.25) construction
  line L250 (-8.3138, 14.4) -> (-10.1325, 11.25) construction
  line L251 (15.8483, -4.95) -> (18.0133, -1.2)
  line L252 (17.6669, 0.6) -> (21.3042, 0.6) construction
  line L253 (10.8253, -3.75) -> (8.6603, 0) construction
  line L254 (8.3138, -6.9) -> (10.1325, -3.75) construction
  line L255 (-8.6603, 15) -> (-10.8253, 11.25) construction
  line L256 (8.6603, 15) -> (10.8253, 11.25) construction
  line L257 (18.0133, -1.2) -> (22.3435, -1.2)
  circle A2 centre (6.4952, 11.25) radius 15.25
  circle A3 centre (6.4952, 11.25) radius 12.5
  line L258 (6.4952, 23.75) -> (6.4952, -1.25) construction
  line L259 (10.4952, 5.75) -> (2.4952, 5.75)
  line L260 (2.4952, 5.75) -> (2.4952, -0.5927)
  line L261 (10.4952, 5.75) -> (10.4952, -0.5927)
  point P0 (19.4856, 11.25)
  point P1 (6.4952, 11.25)
  point P2 (12.9904, 0)
  point P3 (6.4952, -8.7)
  point P4 (6.4952, -6.9)
  point P5 (12.9904, 7.5)
  point P6 (19.4856, 3.75)
  point P7 (-6.4952, 3.75)
  point P8 (12.9904, 7.5)
  point P9 (-6.4952, 11.25)
  point P10 (0, 7.5)
  point P11 (6.4952, 11.25)
  point P12 (0, 15)
  point P13 (12.9904, 0)
  point P14 (0, 7.5)
  point P15 (19.4856, 11.25)
  point P16 (19.4856, 18.75)
  point P17 (6.4952, 26.25)
  point P18 (12.9904, 0)
  point P19 (19.4856, 3.75)
  point P20 (19.4856, 11.25)
  point P21 (12.9904, 15)
  point P22 (6.4952, 18.75)
  point P23 (6.4952, -3.75)
  point P24 (-6.4952, 18.75)
  point P25 (12.9904, 22.5)
  point P26 (-6.4952, 11.25)
  point P27 (-6.4952, 18.75)
  point P28 (6.4952, 3.75)
  point P29 (6.4952, 18.75)
  point P30 (0, 22.5)
  point P31 (6.4952, -3.75)
  point P32 (0, 15)
  point P33 (-6.4952, 3.75)
  point P34 (12.9904, 15)
  point P35 (19.4856, 18.75)
  point P36 (12.9904, 22.5)
  point P37 (6.4952, 26.25)
  point P38 (0, 22.5)
  point P39 (12.9904, 15)
  point P40 (6.4952, 3.75)
  point P41 (6.4952, 5.75)
  dimension "d45" = 7.5
  dimension "d46" = 6.3
  dimension "d47" = 39.9
  dimension "d48" = 30.5
  dimension "d49" = 25
  dimension "d50" = 7
  dimension "d51" = 8
  constraint equal L61 L235
  constraint equal L74 L235
  constraint equal L61 L177
  constraint equal L61 L118
  constraint equal L61 L165
  constraint equal L111 L138
  constraint equal L138 L231
  constraint equal L138 L256
  constraint equal L39 L138
  constraint equal L138 L159
  constraint equal L215 L235
  constraint equal L13 L178
  constraint equal L166 L178
  constraint equal L91 L178
  constraint equal L178 L230
  constraint equal L178 L245
  constraint equal L178 L193
  constraint midpoint L145 L156
  constraint midpoint L9 L118
  constraint midpoint L177 L178
  constraint midpoint L88 L93
  constraint midpoint L130 L165
  constraint midpoint L32 L61
  constraint midpoint L193 L196
  constraint midpoint L50 L53
  constraint midpoint L5 L117
  constraint midpoint L137 L166
  constraint midpoint L11 L114
  constraint midpoint L151 L170
  constraint coincident P18 P13
  constraint midpoint L24 L89
  constraint midpoint L97 L99
  constraint midpoint L163 L168
  constraint midpoint L37 L73
  constraint midpoint L13 L54
  constraint equal L138 L160
  constraint midpoint L132 L160
  constraint coincident P31 P23
  constraint coincident P33 P7
  constraint coincident P14 P10
  constraint coincident P26 P9
  constraint coincident P32 P12
  constraint coincident P11 P1
  constraint coincident P8 P5
  constraint coincident P19 P6
  constraint coincident P20 P15
  constraint coincident P39 P34
  constraint coincident P29 P22
  constraint coincident P27 P24
  constraint coincident P40 P28
  constraint coincident P35 P16
  constraint coincident P36 P25
  constraint coincident P37 P17
  constraint coincident P38 P30
  constraint equal L43 L164
  constraint equal L43 L162
  constraint equal L169 L176
  constraint equal L56 L205
  constraint equal L17 L65
  constraint equal L2 L55
  constraint equal L20 L47
  constraint equal L8 L110
  constraint equal L147 L228
  constraint equal L107 L109
  constraint equal L27 L128
  constraint equal L22 L82
  constraint equal L79 L221
  constraint equal L134 L149
  constraint equal L59 L179
  constraint equal L204 L209
  constraint equal L150 L169
  constraint midpoint P4 L164
  constraint midpoint P3 L167
  constraint coincident P3 A0.centre
  constraint parallel L14 L23
  constraint parallel L133 L167
  constraint parallel L230 L238
  constraint parallel L138 L242
  constraint parallel L243 L251
  constraint parallel L231 L257
  constraint parallel L155 L161
  constraint parallel L7 L129
  constraint parallel L111 L124
  constraint parallel L105 L232
  constraint parallel L64 L86
  constraint parallel L31 L51
  constraint parallel L29 L30
  constraint parallel L136 L141
  constraint parallel L157 L201
  constraint parallel L185 L213
  constraint parallel L139 L146
  constraint parallel L80 L197
  constraint parallel L184 L227
  constraint parallel L69 L210
  constraint parallel L153 L180
  constraint parallel L203 L224
  constraint parallel L206 L212
  constraint parallel L116 L255
  constraint parallel L3 L36
  constraint parallel L0 L1
  constraint parallel L143 L182
  constraint parallel L16 L60
  constraint parallel L42 L85
  constraint parallel L28 L77
  constraint concentric A0 A1
  constraint concentric A2 A3
  constraint horizontal L126
  constraint horizontal L218
  constraint vertical L258
  constraint coincident A3 L258.start
  constraint coincident A3 L258.end
  constraint coincident P11 L258
  constraint vertical L261
  constraint vertical L260
  constraint coincident L258 P41
  constraint midpoint L259 P41
  constraint horizontal L259
  constraint coincident A3 L260.end
  constraint coincident A3 L261.end
  measures "d45" distance of L156 L235
  measures "d46" distance of L95 L237
  measures "d47" distance of L146 L167
  measures "d48" diameter of A2
  measures "d49" diameter of A3
  measures "d50" distance of L258.end L259
  measures "d51" distance of L259.start L259.end
extrude "Extrusion3" add sketch "Skizze2" along normal blind 2 contours L1 L3 L14 L28 L30 L42 L51 L60 L80 L86 L105 L116 L124 L129 L141 L146 L157 L161 L167 L180 L182 L210 L212 L213 L224 L227 L238 L242 L251 L257 | A0 A1 L167 | A2 | A3 L259 L260 L261 | A3 L259 L260 L261
fillet "Abrundung1" radius 0.7 34 edges at (6.4952, 8.7, 1) (6.4952, 9.7579, 1) (6.4952, 11.5579, 1) (2.5548, 6.825, 1) (-0.6928, 4.95, 1) (-3.9404, 3.075, 1) (-7.188, 1.2, 1) (-10.782, -1.275, 1) (-11.1284, -5.625, 1) (-11.1284, -9.375, 1) (-11.1284, -13.125, 1) (-11.1284, -16.875, 1) (-10.782, -21.225, 1) (-7.188, -23.7, 1) (-3.9404, -25.575, 1) (-0.6928, -27.45, 1) (2.5548, -29.325, 1) (6.4952, -31.2, 1) (10.4356, -29.325, 1) (13.6832, -27.45, 1) (16.9308, -25.575, 1) (20.1784, -23.7, 1) (23.7724, -21.225, 1) (24.1188, -16.875, 1) (24.1188, -13.125, 1) (24.1188, -9.375, 1) (24.1188, -5.625, 1) (23.7724, -1.275, 1) (20.1784, 1.2, 1) (16.9308, 3.075, 1) (13.6832, 4.95, 1) (10.4356, 6.825, 1) (6.4952, 8.7, -2) (6.4952, 9.7579, -2) 1 faces at (4.8209, -14.15, -2)
extrude "Extrusion6" cut sketch "Skizze2" along normal blind 1 contours A2 | A3 L259 L260 L261 picked at (6.7664, 3.4255)
fillet "Abrundung2" radius 0.5 108 edges at (9.2232, 2.175, 1) (6.4952, 0.6, 1) (3.7672, 2.175, 1) (3.7672, 5.325, 1) (6.4952, 6.9, 1) (9.2232, 5.325, 1) (10.2624, 1.575, 1) (12.9904, 3.15, 1) (15.7184, 1.575, 1) (15.7184, -1.575, 1) (12.9904, -3.15, 1) (10.2624, -1.575, 1) (16.7576, -5.325, 1) (19.4856, -6.9, 1) (22.2136, -5.325, 1) (22.2136, -2.175, 1) (19.4856, -0.6, 1) (16.7576, -2.175, 1) (22.2136, -9.675, 1) (22.2136, -12.825, 1) (19.4856, -14.4, 1) (16.7576, -12.825, 1) (16.7576, -9.675, 1) (19.4856, -8.1, 1) (15.7184, -9.075, 1) (15.7184, -5.925, 1) (12.9904, -4.35, 1) (10.2624, -5.925, 1) (10.2624, -9.075, 1) (12.9904, -10.65, 1) (9.2232, -5.325, 1) (9.2232, -2.175, 1) (6.4952, -0.6, 1) (3.7672, -2.175, 1) (3.7672, -5.325, 1) (6.4952, -6.9, 1) (2.728, -1.575, 1) (0, -3.15, 1) (-2.728, -1.575, 1) (-2.728, 1.575, 1) (0, 3.15, 1) (2.728, 1.575, 1) (2.728, -9.075, 1) (2.728, -5.925, 1) (0, -10.65, 1) (-2.728, -9.075, 1) (-2.728, -5.925, 1) (0, -4.35, 1) (-3.7672, -5.325, 1) (-3.7672, -2.175, 1) (-6.4952, -0.6, 1) (-9.2232, -2.175, 1) (-9.2232, -5.325, 1) (-6.4952, -6.9, 1) (-3.7672, -9.675, 1) (-3.7672, -12.825, 1) (-6.4952, -14.4, 1) (-9.2232, -12.825, 1) (-9.2232, -9.675, 1) (-6.4952, -8.1, 1) (-3.7672, -20.325, 1) (-3.7672, -17.175, 1) (-6.4952, -15.6, 1) (-9.2232, -17.175, 1) (-9.2232, -20.325, 1) (-6.4952, -21.9, 1) (0, -18.15, 1) (2.728, -16.575, 1) (2.728, -13.425, 1) (0, -11.85, 1) (-2.728, -13.425, 1) (-2.728, -16.575, 1) (2.728, -24.075, 1) (2.728, -20.925, 1) (0, -19.35, 1) (-2.728, -20.925, 1) (-2.728, -24.075, 1) (0, -25.65, 1) (3.7672, -24.675, 1) (6.4952, -23.1, 1) (9.2232, -24.675, 1) (9.2232, -27.825, 1) (6.4952, -29.4, 1) (3.7672, -27.825, 1) (12.9904, -25.65, 1) (15.7184, -24.075, 1) (15.7184, -20.925, 1) (12.9904, -19.35, 1) (10.2624, -20.925, 1) (10.2624, -24.075, 1) (9.2232, -20.325, 1) (6.4952, -21.9, 1) (9.2232, -17.175, 1) (6.4952, -15.6, 1) (3.7672, -17.175, 1) (3.7672, -20.325, 1) (10.2624, -16.575, 1) (12.9904, -18.15, 1) (15.7184, -16.575, 1) (15.7184, -13.425, 1) (12.9904, -11.85, 1) (10.2624, -13.425, 1) (16.7576, -17.175, 1) (16.7576, -20.325, 1) (19.4856, -21.9, 1) (22.2136, -20.325, 1) (22.2136, -17.175, 1) (19.4856, -15.6, 1)